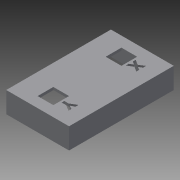
# Autodesk Inventor part: gamebox
Saved by Autodesk Inventor 2015 (Build 190159000, 159)
## iProperties
Created: 2017-03-26
Part Number: gamebox
Material: Generic
Document SubType Name: Modeling
Designer: Tiffany
Density: 1 g/cm^3
Appearance: Default
Author: Tiffany
Autodesk Inventor part; units mm, degrees
ref_plane "YZ Plane" through (0, 0, 0) normal (1, 0, 0) x (0, 1, 0)
ref_plane "XZ Plane" through (0, 0, 0) normal (0, 1, 0) x (-1, 0, 0)
ref_plane "XY Plane" through (0, 0, 0) normal (0, 0, 1) x (1, 0, 0)
sketch "Sketch1" plane through (0, 0, 0) normal (0, 1, 0) x (-1, 0, 0)
  line L0 (0, 0) -> (76.2, 0)
  line L1 (76.2, 0) -> (76.2, -127)
  line L2 (76.2, -127) -> (0, -127)
  line L3 (0, -127) -> (0, 0)
  dimension "d0" = 76.2
  dimension "d1" = 127
  constraints: 8 end point, 2 parallel, 1 horizontal, 1 perpendicular
  measures "d0" distance of L1.end L2.end
  measures "d1" distance of L0.end L1.end
extrude "Extrusion1" add sketch "Sketch1" along normal blind 25.4
sketch "Sketch2" plane through (0, 0, 0) normal (0, -1, 0) x (1, 0, 0)
  line L0 (-3.1691, -3.1691) -> (-72.8902, -3.1691)
  line L1 (-72.8902, -3.1691) -> (-72.8902, -123.5964)
  line L2 (-72.8902, -123.5964) -> (-3.1691, -123.5964)
  line L3 (-3.1691, -123.5964) -> (-3.1691, -3.1691)
  point P0 (0, 0)
  constraints: 8 end point, 2 parallel, 1 horizontal, 1 perpendicular
extrude "Extrusion2" cut sketch "Sketch2" against normal blind 22.225
sketch "Sketch3" plane through (0, 25.4, 0) normal (0, 1, 0) x (1, 0, 0)
  line L0 (-50.8, 12.7) -> (-31.75, 12.7)
  line L1 (-31.75, 12.7) -> (-31.75, 31.75)
  line L2 (-31.75, 31.75) -> (-50.8, 31.75)
  line L3 (-50.8, 31.75) -> (-50.8, 12.7)
  line L4 (-50.8, 95.25) -> (-31.75, 95.25)
  line L5 (-31.75, 95.25) -> (-31.75, 114.3)
  line L6 (-31.75, 114.3) -> (-50.8, 114.3)
  line L7 (-50.8, 114.3) -> (-50.8, 95.25)
  line L8 (-76.2, 127) -> (-76.2, 0) projected
  line L9 (-76.2, 0) -> (0, 0) projected
  line L10 (0, 127) -> (-76.2, 127) projected
  dimension "d6" = 19.05
  dimension "d7" = 19.05
  dimension "d8" = 25.4
  dimension "d9" = 25.4
  dimension "d10" = 19.05
  dimension "d11" = 19.05
  dimension "d12" = 12.7
  dimension "d13" = 12.7
  constraints: 16 end point, 4 parallel, 2 horizontal, 2 perpendicular
  measures "d6" distance between parallel lines of L2 L0
  measures "d7" distance between parallel lines of L6 L4
  measures "d8" distance between parallel lines of L8 L3
  measures "d9" distance between parallel lines of L8 L7
  measures "d10" distance of L1.end L2.end
  measures "d11" distance of L4.start L4.end
  measures "d12" distance between parallel lines of L9 L0
  measures "d13" distance between parallel lines of L10 L6
extrude "Extrusion3" cut sketch "Sketch3" against normal blind 22.225
sketch "Sketch4" plane through (0, 25.4, 0) normal (0, 1, 0) x (1, 0, 0)
  line L0 (-13.7708, 110.3112) -> (-13.7708, 97.845) construction
  line L1 (-13.7708, 97.845) -> (-32.3251, 97.845) construction
  line L2 (-32.3251, 97.845) -> (-32.3251, 110.3112) construction
  line L3 (-32.3251, 110.3112) -> (-13.7708, 110.3112) construction
  line L4 (-12.0313, 30.7306) -> (-12.0313, 13.191) construction
  line L5 (-12.0313, 13.191) -> (-34.0646, 13.191) construction
  line L6 (-34.0646, 13.191) -> (-34.0646, 30.7306) construction
  line L7 (-34.0646, 30.7306) -> (-12.0313, 30.7306) construction
  line L8 (-29.3979, 98.0986) -> (-29.3979, 101.783)
  line L9 (-29.3979, 101.783) -> (-25.3533, 104.2325)
  line L10 (-25.3533, 104.2325) -> (-29.3979, 106.7333)
  line L11 (-29.3979, 106.7333) -> (-29.3979, 110.2634)
  line L12 (-29.3979, 110.2634) -> (-23.0068, 106.1364)
  line L13 (-23.0068, 106.1364) -> (-16.6979, 110.0987)
  line L14 (-16.6979, 110.0987) -> (-16.6979, 106.4143)
  line L15 (-16.6979, 106.4143) -> (-20.5367, 104.1192)
  line L16 (-20.5367, 104.1192) -> (-16.6979, 101.7624)
  line L17 (-16.6979, 101.7624) -> (-16.6979, 98.2324)
  line L18 (-16.6979, 98.2324) -> (-22.873, 102.2153)
  line L19 (-22.873, 102.2153) -> (-29.3979, 98.0986)
  line L20 (-16.6979, 16.0996) -> (-24.0977, 20.4839)
  line L21 (-24.0977, 20.4839) -> (-29.3979, 20.4839)
  line L22 (-29.3979, 20.4839) -> (-29.3979, 23.6743)
  line L23 (-29.3979, 23.6743) -> (-24.2521, 23.6743)
  line L24 (-24.2521, 23.6743) -> (-16.6979, 28.1307)
  line L25 (-16.6979, 28.1307) -> (-16.6979, 24.4977)
  line L26 (-16.6979, 24.4977) -> (-21.2263, 22.0174)
  line L27 (-21.2263, 22.0174) -> (-16.6979, 19.6194)
  line L28 (-16.6979, 19.6194) -> (-16.6979, 16.0996)
  point P0 (0, 0)
  constraints: 4 other
extrude "Extrusion4" cut sketch "Sketch4" against normal blind 25.4
body "Solid1"
